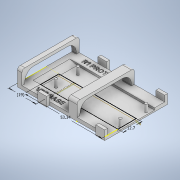
# Autodesk Inventor part: R1 Proto V10 Base
Saved by Autodesk Inventor 2021 (Build 250183000, 183)
## iProperties
Created: 2020-06-07
Part Number: R1 Proto V10 Base
Material: Generic
Document SubType Name: Modeling
Designer: andre
Density: 1 g/cm^3
Appearance: Default
Author: andre
## iProperties of the stored document _3DPrint.ipt
Created: 2020-06-07
Part Number: _3DPrint
Material: Generic
Document SubType Name: Modeling
Designer: andre
Density: 1 g/cm^3
Appearance: Default
Author: andre
Autodesk Inventor part; units mm, degrees
ref_plane "YZ Plane" through (0, 0, 0) normal (1, 0, 0) x (0, 1, 0)
ref_plane "XZ Plane" through (0, 0, 0) normal (0, 1, 0) x (-1, 0, 0)
ref_plane "XY Plane" through (0, 0, 0) normal (0, 0, 1) x (1, 0, 0)
sketch "Sketch1" plane through (0, 0, 0) normal (0, 1, 0) x (-1, 0, 0)
  line L0 (0, 0) -> (62, 0)
  line L1 (62, 0) -> (62, -19.7)
  line L2 (62, -19.7) -> (0, -19.7)
  line L3 (0, -19.7) -> (0, 0)
  dimension "d5" = 62
  dimension "d6" = 19.7
  constraints: 8 end point, 2 parallel, 1 horizontal, 1 perpendicular
  measures "d5" distance of L1.end L2.end
  measures "d6" distance of L0.end L1.end
extrude "Extrusion1" add sketch "Sketch1" along normal blind 2.4
sketch "Sketch2" plane through (0, 2.4, 0) normal (0, 1, 0) x (1, 0, 0)
  point P0 (0, 0)
sketch "Sketch3" plane through (-62, 0, 0) normal (0, 0, 1) x (1, 0, 0)
  line L0 (62, 2.4) -> (0, 2.4) projected
  line L1 (62, 0) -> (0, 0) projected
  line L2 (62, 2.4) -> (56, 2.4)
  line L3 (56, 2.4) -> (56, 0)
  line L4 (56, 0) -> (62, 0)
  line L5 (62, 0) -> (62, 2.4)
  line L6 (22, 2.4) -> (22, 0) construction
  line L7 (22, 2.4) -> (16, 2.4)
  line L8 (16, 2.4) -> (16, 0)
  line L9 (16, 0) -> (22, 0)
  line L10 (22, 0) -> (22, 2.4)
  point P0 (62, 0)
  point P1 (22, 0)
  dimension "d9" = 6
  dimension "d13" = 6
  dimension "d14" = 34
  constraints: 18 end point, 4 parallel, 4 point on line, 3 perpendicular, 2 horizontal
  measures "d9" distance of L4.end L3.end
  measures "d13" distance of L9.end L8.end
  measures "d14" distance between parallel lines of L3 L6
extrude "Extrusion2" add sketch "Sketch3" along normal blind 2 contours L5 L1 L3 L0 | L10 L1 L8 L0
ref_plane "Work Plane1" through (0, 0, -19.7) normal (0, 0, -1) x (-1, 0, 0)
sketch "Sketch4" plane through (0, 2.4, 0) normal (0, 1, 0) x (1, 0, 0)
  line L0 (-6, -2) -> (0, -2) projected
  line L1 (-6, -2) -> (0, -2)
  line L2 (0, -2) -> (0, 0)
  line L3 (0, 0) -> (-6, 0)
  line L4 (-6, 0) -> (-6, -2)
  line L5 (-46, -2) -> (-40, -2) projected
  line L6 (-40, 0) -> (-40, -2) projected
  line L7 (-46, -2) -> (-40, -2)
  line L8 (-40, -2) -> (-40, 0)
  line L9 (-40, 0) -> (-46, 0)
  line L10 (-46, 0) -> (-46, -2)
  constraints: 16 end point, 4 parallel, 2 horizontal, 2 perpendicular
extrude "Extrusion3" add sketch "Sketch4" along normal blind 4
sketch "Sketch5" plane through (0, 2.4, 0) normal (0, 1, 0) x (1, 0, 0)
  point P0 (0, 0)
sketch "Sketch6" plane through (0, 2.4, 0) normal (0, 1, 0) x (1, 0, 0)
  line L0 (0, 19.7) -> (-62, 19.7) projected
  line L1 (-40, 0) -> (-6, 0) projected
  line L2 (-21, 19.7) -> (-27, 19.7)
  line L3 (-27, 19.7) -> (-27, 0)
  line L4 (-27, 0) -> (-21, 0)
  line L5 (-21, 0) -> (-21, 19.7)
  line L6 (0, 19.7) -> (0, 0) projected
  dimension "d18" = 6
  dimension "d19" = 21
  constraints: 8 end point, 2 parallel, 2 point on line, 1 horizontal, 1 perpendicular
  measures "d18" distance of L4.end L3.end
  measures "d19" distance between parallel lines of L6 L5
extrude "Extrusion4" add sketch "Sketch6" along normal blind 9.6
sketch "Sketch7" plane through (-21, 2.4, 0) normal (1, 0, 0) x (0, 0, -1)
  point P0 (0, -2.4)
sketch "Sketch8" plane through (-21, 2.4, 0) normal (1, 0, 0) x (0, 0, -1)
  line L0 (19.7, 0) -> (19.7, 9.6) projected
  line L1 (19.7, 0) -> (2, 0)
  line L2 (2, 0) -> (2, 7.6)
  line L3 (2, 7.6) -> (19.7, 7.6)
  line L4 (19.7, 7.6) -> (19.7, 0)
  line L5 (0, 0) -> (0, 9.6) projected
  line L6 (19.7, 0) -> (0, 0) projected
  line L7 (0, 9.6) -> (19.7, 9.6) projected
  point P0 (0, -2.4)
  dimension "d22" = 19.7
  dimension "d23" = 9.6
  dimension "d24" = 17.7
  dimension "d25" = 7.6
  constraints: 8 end point, 2 parallel, 1 horizontal, 1 perpendicular
  measures "d22" distance between parallel lines of L0 L5
  measures "d23" distance between parallel lines of L6 L7
  measures "d24" distance between parallel lines of L0 L2
  measures "d25" distance between parallel lines of L1 L3
extrude "Extrusion5" cut sketch "Sketch8" against normal blind 37.6 contours L1 L2 L3 L0
sketch "Sketch9" plane through (0, 2.4, 0) normal (0, 1, 0) x (1, 0, 0)
  line L0 (-40, 0) -> (-46, 0) construction
  line L1 (-43, 0) -> (-43, 19.7) construction
  line L2 (0, 19.7) -> (-62, 19.7) construction
  line L3 (-62, 19.7) -> (-62, 0) projected
  point P0 (0, 0)
  dimension "d30" = 19
  constraints: 2 end point, 1 midpoint, 1 point on line, 1 vertical
  measures "d30" distance between parallel lines of L3 L1
ref_plane "Work Plane2" through (-43, 0, -19.7) normal (-1, 0, 0) x (0, 0, 1)
mirror "Mirror2" about plane through (-43, 0, -19.7) normal (-1, 0, 0) of "Extrusion4", "Extrusion5"
sketch "Sketch12" plane through (0, 2.4, 0) normal (0, 1, 0) x (1, 0, 0)
  line L0 (0, 19.7) -> (0, -2) projected
  line L1 (0, 19.7) -> (-53.34, 19.7)
  line L2 (-53.34, 19.7) -> (-53.34, 7)
  line L3 (-53.34, 7) -> (0, 7)
  line L4 (0, 7) -> (0, 19.7)
  point P0 (0, 0)
  point P1 (0, 7)
  dimension "d41" = 53.34
  dimension "d42" = 12.7
  constraints: 8 end point, 2 parallel, 1 horizontal, 1 perpendicular
  measures "d41" distance between parallel lines of L2 L0
  measures "d42" distance between parallel lines of L1 L3
extrude "Extrusion8" cut sketch "Sketch12" against normal blind 1.4
fillet "Fillet3" radius 2 2 edges at (-62, 12, 0) (-24, 12, 0) curvature continuous yes
fillet "Fillet4" radius 7 2 edges at (-62, 10, -2) (-24, 10, -2) curvature continuous yes
sketch "Sketch13" plane through (0, 1, 0) normal (0, 1, 0) x (1, 0, 0)
  circle A0 centre (-1.9751, 10.81) radius 0.9
  circle A1 centre (-47.6951, 12.1417) radius 0.9
  line L0 (-53.34, 19.7) -> (0, 19.7) projected
  point P0 (0, 0)
  dimension "d48" = 1.8
  dimension "d49" = 1.8
  dimension "d50" = 45.72
  dimension "d51" = 8.89
  constraints: 2 centre point
  measures "d48" diameter of A0
  measures "d49" diameter of A1
  measures "d50" horizontal distance of A1.centre A0.centre
  measures "d51" distance from line of L0 A0.centre
extrude "Extrusion9" add sketch "Sketch13" along normal blind 5
mirror "Mirror3" about plane through (0, 0, -19.7) normal (0, 0, -1) of "Extrusion4", "Extrusion5", "Mirror2", "Fillet4", "Fillet3", "Extrusion1", "Extrusion3", "Extrusion2", "Extrusion9", "Extrusion8"
sketch "Sketch14" plane through (-62, 0, 0) normal (-1, 0, 0) x (0, 0, 1)
  line L0 (-58.5888, -16.4354) -> (8.8289, -16.4354)
  line L1 (8.8289, -16.4354) -> (8.8289, 25.7982)
  line L2 (8.8289, 25.7982) -> (-58.5888, 25.7982)
  line L3 (-58.5888, 25.7982) -> (-58.5888, -16.4354)
  point P0 (0, 0)
  constraints: 8 end point, 2 parallel, 1 horizontal, 1 perpendicular
extrude "Extrusion10" cut sketch "Sketch14" along normal blind 5
chamfer "Chamfer1" distance 5 distance2 1.4 1 edges at (-53.34, 2.4, -19.7) measured on face at (-53.84, 2.4, -19.7)
sketch "Sketch15" plane through (0, 2.4, 0) normal (0, 1, 0) x (1, 0, 0)
  line L0 (-57, 38.4) -> (-29, 38.4) construction
  line L1 (-29, 38.4) -> (-29, 33.4) construction
  line L2 (-29, 33.4) -> (-57, 33.4) construction
  line L3 (-57, 33.4) -> (-57, 38.4) construction
  line L4 (-59, 37.4) -> (-59, 2) projected
  line L5 (-27, 2) -> (-27, 37.4) projected
  line L6 (-59, 39.4) -> (-46, 39.4) projected
  line L7 (-58.34, 32.4) -> (0, 32.4) projected
  line L8 (-57, 6) -> (-29, 6) construction
  line L9 (-29, 6) -> (-29, 1) construction
  line L10 (-29, 1) -> (-57, 1) construction
  line L11 (-57, 1) -> (-57, 6) construction
  line L12 (0, 7) -> (-58.34, 7) projected
  line L13 (-59, 0) -> (-46, 0) projected
  spline S0 degree 2 poles (-51.0157, 2) (-50.8394, 2) (-50.6147, 2.1691) (-50.5495, 2.3527) knots 0 0 0 1 2 2 2
  line L14 (-50.5495, 2.3527) -> (-49.7307, 4.5556)
  spline S1 degree 2 poles (-49.7307, 4.5556) (-49.7017, 4.6377) (-49.7017, 4.7174) knots 0 0 0 1 1 1
  spline S2 degree 2 poles (-49.7017, 4.7174) (-49.7041, 4.8454) (-49.8732, 4.9976) (-50.0157, 5) knots 0 0 0 1 2 2 2
  spline S3 degree 2 poles (-50.0157, 5) (-50.1341, 5) (-50.279, 4.8865) (-50.3176, 4.7657) knots 0 0 0 1 2 2 2
  line L15 (-50.3176, 4.7657) -> (-50.9988, 2.6691)
  line L16 (-50.9988, 2.6691) -> (-51.0133, 2.6691)
  line L17 (-51.0133, 2.6691) -> (-51.6969, 4.7585)
  spline S4 degree 2 poles (-51.6969, 4.7585) (-51.7331, 4.8841) (-51.8853, 5) (-52.0085, 5) knots 0 0 0 1 2 2 2
  spline S5 degree 2 poles (-52.0085, 5) (-52.1558, 4.9976) (-52.3273, 4.8406) (-52.3297, 4.7101) knots 0 0 0 1 2 2 2
  spline S6 degree 2 poles (-52.3297, 4.7101) (-52.3297, 4.6232) (-52.3007, 4.5386) knots 0 0 0 1 1 1
  line L18 (-52.3007, 4.5386) -> (-51.4867, 2.3551)
  spline S7 degree 2 poles (-51.4867, 2.3551) (-51.4215, 2.1691) (-51.1944, 2) (-51.0157, 2) knots 0 0 0 1 2 2 2
  spline S8 degree 2 poles (-48.3708, 1.9952) (-48.2331, 1.9976) (-48.0713, 2.1618) (-48.0688, 2.3019) knots 0 0 0 1 2 2 2
  line L19 (-48.0688, 2.3019) -> (-48.0688, 4.6618)
  spline S9 degree 2 poles (-48.0688, 4.6618) (-48.0713, 4.8213) (-48.2524, 5.0024) (-48.4167, 5.0048) knots 0 0 0 1 2 2 2
  spline S10 degree 2 poles (-48.4167, 5.0048) (-48.5085, 5.0048) (-48.6751, 4.9589) (-48.779, 4.8889) knots 0 0 0 1 2 2 2
  line L20 (-48.779, 4.8889) -> (-49.3587, 4.4879)
  spline S11 degree 2 poles (-49.3587, 4.4879) (-49.4287, 4.4372) (-49.4915, 4.3285) (-49.4915, 4.2585) knots 0 0 0 1 2 2 2
  spline S12 degree 2 poles (-49.4915, 4.2585) (-49.4891, 4.1594) (-49.3708, 4.0411) (-49.2766, 4.0411) knots 0 0 0 1 2 2 2
  spline S13 degree 2 poles (-49.2766, 4.0411) (-49.2307, 4.0411) (-49.1558, 4.0652) (-49.1147, 4.0942) knots 0 0 0 1 2 2 2
  line L21 (-49.1147, 4.0942) -> (-48.6872, 4.3937)
  line L22 (-48.6872, 4.3937) -> (-48.6751, 4.3937)
  line L23 (-48.6751, 4.3937) -> (-48.6751, 2.3019)
  spline S14 degree 2 poles (-48.6751, 2.3019) (-48.6727, 2.1618) (-48.5085, 1.9976) (-48.3708, 1.9952) knots 0 0 0 1 2 2 2
  spline S15 degree 2 poles (-46.2597, 1.9734) (-45.8877, 1.9758) (-45.3563, 2.3478) (-45.0713, 3.0314) (-45.0688, 3.5072) knots 0 0 0 1 2 3 3 3
  spline S16 degree 2 poles (-45.0688, 3.5072) (-45.0713, 3.9807) (-45.3563, 4.6594) (-45.8901, 5.0242) (-46.2597, 5.0266) knots 0 0 0 1 2 3 3 3
  spline S17 degree 2 poles (-46.2597, 5.0266) (-46.6292, 5.0242) (-47.163, 4.657) (-47.4505, 3.9783) (-47.4505, 3.5048) knots 0 0 0 1 2 3 3 3
  spline S18 degree 2 poles (-47.4505, 3.5048) (-47.4505, 3.029) (-47.163, 2.3454) (-46.6316, 1.9758) (-46.2597, 1.9734) knots 0 0 0 1 2 3 3 3
  spline S19 degree 2 poles (-46.2597, 2.4638) (-46.5326, 2.4662) (-46.8273, 3) (-46.8297, 3.5048) knots 0 0 0 1 2 2 2
  spline S20 degree 2 poles (-46.8297, 3.5048) (-46.8273, 4.0048) (-46.5278, 4.5338) (-46.2597, 4.5362) knots 0 0 0 1 2 2 2
  spline S21 degree 2 poles (-46.2597, 4.5362) (-45.9891, 4.5338) (-45.692, 4.0048) (-45.6896, 3.5048) knots 0 0 0 1 2 2 2
  spline S22 degree 2 poles (-45.6896, 3.5048) (-45.692, 3) (-45.9867, 2.4662) (-46.2597, 2.4638) knots 0 0 0 1 2 2 2
  line L24 (-43.535, 2.0386) -> (-42.5471, 2.0386)
  spline S23 degree 2 poles (-42.5471, 2.0386) (-42.0737, 2.0435) (-41.5423, 2.4855) (-41.5374, 2.8744) knots 0 0 0 1 2 2 2
  spline S24 degree 2 poles (-41.5374, 2.8744) (-41.5423, 3.1691) (-41.9215, 3.5531) (-42.2258, 3.5821) knots 0 0 0 1 2 2 2
  line L25 (-42.2258, 3.5821) -> (-42.2258, 3.5966)
  spline S25 degree 2 poles (-42.2258, 3.5966) (-41.9867, 3.6377) (-41.6824, 3.9855) (-41.6775, 4.2319) knots 0 0 0 1 2 2 2
  spline S26 degree 2 poles (-41.6775, 4.2319) (-41.68, 4.57) (-42.1534, 4.9565) (-42.5688, 4.9589) knots 0 0 0 1 2 2 2
  line L26 (-42.5688, 4.9589) -> (-43.535, 4.9589)
  spline S27 degree 2 poles (-43.535, 4.9589) (-43.68, 4.9589) (-43.8394, 4.7923) (-43.8394, 4.6425) knots 0 0 0 1 2 2 2
  line L27 (-43.8394, 4.6425) -> (-43.8394, 2.3575)
  spline S28 degree 2 poles (-43.8394, 2.3575) (-43.8394, 2.2053) (-43.68, 2.0386) (-43.535, 2.0386) knots 0 0 0 1 2 2 2
  line L28 (-43.2283, 2.4952) -> (-43.2283, 3.343)
  line L29 (-43.2283, 3.343) -> (-42.7162, 3.343)
  spline S29 degree 2 poles (-42.7162, 3.343) (-42.4457, 3.3406) (-42.1606, 3.128) (-42.1606, 2.9227) knots 0 0 0 1 2 2 2
  spline S30 degree 2 poles (-42.1606, 2.9227) (-42.1606, 2.7126) (-42.4384, 2.4952) (-42.7041, 2.4952) knots 0 0 0 1 2 2 2
  line L30 (-42.7041, 2.4952) -> (-43.2283, 2.4952)
  line L31 (-43.2283, 3.744) -> (-43.2283, 4.5048)
  line L32 (-43.2283, 4.5048) -> (-42.7283, 4.5048)
  spline S31 degree 2 poles (-42.7283, 4.5048) (-42.5109, 4.5024) (-42.279, 4.3116) (-42.279, 4.1353) knots 0 0 0 1 2 2 2
  spline S32 degree 2 poles (-42.279, 4.1353) (-42.279, 3.9493) (-42.5447, 3.7464) (-42.7911, 3.744) knots 0 0 0 1 2 2 2
  line L33 (-42.7911, 3.744) -> (-43.2283, 3.744)
  spline S33 degree 2 poles (-40.994, 2) (-40.8732, 2) (-40.7258, 2.1304) (-40.6848, 2.2754) knots 0 0 0 1 2 2 2
  line L34 (-40.6848, 2.2754) -> (-40.5302, 2.7319)
  line L35 (-40.5302, 2.7319) -> (-39.4771, 2.7319)
  line L36 (-39.4771, 2.7319) -> (-39.3225, 2.2705)
  spline S34 degree 2 poles (-39.3225, 2.2705) (-39.2814, 2.128) (-39.1316, 2) (-39.0036, 2) knots 0 0 0 1 2 2 2
  spline S35 degree 2 poles (-39.0036, 2) (-38.8684, 2.0024) (-38.7017, 2.1594) (-38.6993, 2.2874) knots 0 0 0 1 2 2 2
  spline S36 degree 2 poles (-38.6993, 2.2874) (-38.6993, 2.3333) (-38.7162, 2.4227) (-38.7379, 2.4831) knots 0 0 0 1 2 2 2
  line L37 (-38.7379, 2.4831) -> (-39.5399, 4.6546)
  spline S37 degree 2 poles (-39.5399, 4.6546) (-39.6027, 4.8333) (-39.8273, 5) (-40.006, 5) knots 0 0 0 1 2 2 2
  spline S38 degree 2 poles (-40.006, 5) (-40.1775, 5) (-40.4022, 4.8309) (-40.465, 4.6546) knots 0 0 0 1 2 2 2
  line L38 (-40.465, 4.6546) -> (-41.2621, 2.4831)
  spline S39 degree 2 poles (-41.2621, 2.4831) (-41.2838, 2.4251) (-41.3031, 2.3261) (-41.3031, 2.2874) knots 0 0 0 1 2 2 2
  spline S40 degree 2 poles (-41.3031, 2.2874) (-41.3031, 2.1546) (-41.1389, 2.0024) (-40.994, 2) knots 0 0 0 1 2 2 2
  line L39 (-40.3973, 3.2053) -> (-40.0181, 4.401)
  line L40 (-40.0181, 4.401) -> (-40.0036, 4.401)
  line L41 (-40.0036, 4.401) -> (-39.6171, 3.2053)
  line L42 (-39.6171, 3.2053) -> (-40.3973, 3.2053)
  spline S41 degree 2 poles (-37.2597, 1.9903) (-36.7089, 1.9952) (-36.0882, 2.4879) (-36.0833, 2.9203) knots 0 0 0 1 2 2 2
  spline S42 degree 2 poles (-36.0833, 2.9203) (-36.0809, 3.2512) (-36.5085, 3.6473) (-36.9698, 3.7367) knots 0 0 0 1 2 2 2
  line L43 (-36.9698, 3.7367) -> (-37.279, 3.7995)
  spline S43 degree 2 poles (-37.279, 3.7995) (-37.535, 3.8502) (-37.7669, 4.0266) (-37.7645, 4.1594) knots 0 0 0 1 2 2 2
  spline S44 degree 2 poles (-37.7645, 4.1594) (-37.7597, 4.3237) (-37.4915, 4.5145) (-37.2621, 4.5169) knots 0 0 0 1 2 2 2
  spline S45 degree 2 poles (-37.2621, 4.5169) (-37.0737, 4.5169) (-36.7983, 4.3696) (-36.7258, 4.2053) knots 0 0 0 1 2 2 2
  spline S46 degree 2 poles (-36.7258, 4.2053) (-36.6751, 4.1111) (-36.535, 4.0242) (-36.4336, 4.0242) knots 0 0 0 1 2 2 2
  spline S47 degree 2 poles (-36.4336, 4.0242) (-36.3152, 4.0266) (-36.1751, 4.1594) (-36.1727, 4.2681) knots 0 0 0 1 2 2 2
  spline S48 degree 2 poles (-36.1727, 4.2681) (-36.1727, 4.3092) (-36.1848, 4.3744) (-36.1944, 4.4058) knots 0 0 0 1 2 2 2
  spline S49 degree 2 poles (-36.1944, 4.4058) (-36.2959, 4.6932) (-36.8563, 5.0072) (-37.2621, 5.0097) knots 0 0 0 1 2 2 2
  spline S50 degree 2 poles (-37.2621, 5.0097) (-37.5882, 5.0072) (-38.0906, 4.7874) (-38.3732, 4.3913) (-38.378, 4.1208) knots 0 0 0 1 2 3 3 3
  spline S51 degree 2 poles (-38.378, 4.1208) (-38.378, 3.7947) (-37.9457, 3.3792) (-37.5085, 3.2923) knots 0 0 0 1 2 2 2
  line L44 (-37.5085, 3.2923) -> (-37.1993, 3.2319)
  spline S52 degree 2 poles (-37.1993, 3.2319) (-36.9263, 3.1763) (-36.692, 2.9976) (-36.6944, 2.8551) knots 0 0 0 1 2 2 2
  spline S53 degree 2 poles (-36.6944, 2.8551) (-36.6993, 2.6908) (-36.9964, 2.4855) (-37.2452, 2.4831) knots 0 0 0 1 2 2 2
  spline S54 degree 2 poles (-37.2452, 2.4831) (-37.4577, 2.4807) (-37.7742, 2.6401) (-37.849, 2.8068) knots 0 0 0 1 2 2 2
  spline S55 degree 2 poles (-37.849, 2.8068) (-37.9022, 2.901) (-38.0374, 2.9855) (-38.1292, 2.9831) knots 0 0 0 1 2 2 2
  spline S56 degree 2 poles (-38.1292, 2.9831) (-38.25, 2.9831) (-38.3973, 2.8382) (-38.3998, 2.715) knots 0 0 0 1 2 2 2
  spline S57 degree 2 poles (-38.3998, 2.715) (-38.3998, 2.6739) (-38.3829, 2.5894) (-38.3659, 2.5507) knots 0 0 0 1 2 2 2
  spline S58 degree 2 poles (-38.3659, 2.5507) (-38.2766, 2.3068) (-37.7138, 1.9952) (-37.2597, 1.9903) knots 0 0 0 1 2 2 2
  line L45 (-35.407, 2.0386) -> (-34.0181, 2.0386)
  spline S59 degree 2 poles (-34.0181, 2.0386) (-33.8901, 2.0386) (-33.7428, 2.1715) (-33.7403, 2.2923) knots 0 0 0 1 2 2 2
  spline S60 degree 2 poles (-33.7403, 2.2923) (-33.7428, 2.4106) (-33.8925, 2.5435) (-34.0181, 2.5435) knots 0 0 0 1 2 2 2
  line L46 (-34.0181, 2.5435) -> (-35.1002, 2.5435)
  line L47 (-35.1002, 2.5435) -> (-35.1002, 3.2826)
  line L48 (-35.1002, 3.2826) -> (-34.0713, 3.2826)
  spline S61 degree 2 poles (-34.0713, 3.2826) (-33.9529, 3.2826) (-33.8176, 3.4058) (-33.8152, 3.5169) knots 0 0 0 1 2 2 2
  spline S62 degree 2 poles (-33.8152, 3.5169) (-33.8176, 3.6256) (-33.9553, 3.7512) (-34.0713, 3.7512) knots 0 0 0 1 2 2 2
  line L49 (-34.0713, 3.7512) -> (-35.1002, 3.7512)
  line L50 (-35.1002, 3.7512) -> (-35.1002, 4.4541)
  line L51 (-35.1002, 4.4541) -> (-34.0181, 4.4541)
  spline S63 degree 2 poles (-34.0181, 4.4541) (-33.8925, 4.4541) (-33.7428, 4.587) (-33.7403, 4.7053) knots 0 0 0 1 2 2 2
  spline S64 degree 2 poles (-33.7403, 4.7053) (-33.7428, 4.8261) (-33.8901, 4.9589) (-34.0181, 4.9589) knots 0 0 0 1 2 2 2
  line L52 (-34.0181, 4.9589) -> (-35.407, 4.9589)
  spline S65 degree 2 poles (-35.407, 4.9589) (-35.5519, 4.9589) (-35.7114, 4.7923) (-35.7114, 4.6425) knots 0 0 0 1 2 2 2
  line L53 (-35.7114, 4.6425) -> (-35.7114, 2.3575)
  spline S66 degree 2 poles (-35.7114, 2.3575) (-35.7114, 2.2053) (-35.5519, 2.0386) (-35.407, 2.0386) knots 0 0 0 1 2 2 2
  spline S67 degree 2 poles (-52.1534, 34.3952) (-52.0085, 34.3976) (-51.849, 34.5618) (-51.8466, 34.714) knots 0 0 0 1 2 2 2
  line L54 (-51.8466, 34.714) -> (-51.8466, 35.5063)
  line L55 (-51.8466, 35.5063) -> (-51.3273, 35.5063)
  line L56 (-51.3273, 35.5063) -> (-50.8418, 34.6271)
  spline S68 degree 2 poles (-50.8418, 34.6271) (-50.7717, 34.4966) (-50.6365, 34.3928) (-50.5302, 34.3952) knots 0 0 0 1 2 2 2
  spline S69 degree 2 poles (-50.5302, 34.3952) (-50.3949, 34.3976) (-50.2258, 34.5522) (-50.221, 34.6754) knots 0 0 0 1 2 2 2
  spline S70 degree 2 poles (-50.221, 34.6754) (-50.221, 34.7261) (-50.25, 34.8227) (-50.2862, 34.8855) knots 0 0 0 1 2 2 2
  line L57 (-50.2862, 34.8855) -> (-50.7089, 35.615)
  spline S71 degree 2 poles (-50.7089, 35.615) (-50.465, 35.7213) (-50.2065, 36.1512) (-50.2065, 36.429) knots 0 0 0 1 2 2 2
  spline S72 degree 2 poles (-50.2065, 36.429) (-50.2089, 36.8662) (-50.7548, 37.3541) (-51.2621, 37.3589) knots 0 0 0 1 2 2 2
  line L58 (-51.2621, 37.3589) -> (-52.1534, 37.3589)
  spline S73 degree 2 poles (-52.1534, 37.3589) (-52.2983, 37.3589) (-52.4577, 37.1923) (-52.4577, 37.0425) knots 0 0 0 1 2 2 2
  line L59 (-52.4577, 37.0425) -> (-52.4577, 34.714)
  spline S74 degree 2 poles (-52.4577, 34.714) (-52.4577, 34.5618) (-52.2983, 34.3976) (-52.1534, 34.3952) knots 0 0 0 1 2 2 2
  line L60 (-51.8466, 35.9507) -> (-51.8466, 36.8807)
  line L61 (-51.8466, 36.8807) -> (-51.3273, 36.8807)
  spline S75 degree 2 poles (-51.3273, 36.8807) (-51.0978, 36.8783) (-50.837, 36.6319) (-50.8345, 36.4169) knots 0 0 0 1 2 2 2
  spline S76 degree 2 poles (-50.8345, 36.4169) (-50.8345, 36.1971) (-51.0882, 35.9531) (-51.3225, 35.9507) knots 0 0 0 1 2 2 2
  line L62 (-51.3225, 35.9507) -> (-51.8466, 35.9507)
  spline S77 degree 2 poles (-48.8104, 34.3952) (-48.6727, 34.3976) (-48.5109, 34.5618) (-48.5085, 34.7019) knots 0 0 0 1 2 2 2
  line L63 (-48.5085, 34.7019) -> (-48.5085, 37.0618)
  spline S78 degree 2 poles (-48.5085, 37.0618) (-48.5109, 37.2213) (-48.692, 37.4024) (-48.8563, 37.4048) knots 0 0 0 1 2 2 2
  spline S79 degree 2 poles (-48.8563, 37.4048) (-48.9481, 37.4048) (-49.1147, 37.3589) (-49.2186, 37.2889) knots 0 0 0 1 2 2 2
  line L64 (-49.2186, 37.2889) -> (-49.7983, 36.8879)
  spline S80 degree 2 poles (-49.7983, 36.8879) (-49.8684, 36.8372) (-49.9312, 36.7285) (-49.9312, 36.6585) knots 0 0 0 1 2 2 2
  spline S81 degree 2 poles (-49.9312, 36.6585) (-49.9287, 36.5594) (-49.8104, 36.4411) (-49.7162, 36.4411) knots 0 0 0 1 2 2 2
  spline S82 degree 2 poles (-49.7162, 36.4411) (-49.6703, 36.4411) (-49.5954, 36.4652) (-49.5543, 36.4942) knots 0 0 0 1 2 2 2
  line L65 (-49.5543, 36.4942) -> (-49.1268, 36.7937)
  line L66 (-49.1268, 36.7937) -> (-49.1147, 36.7937)
  line L67 (-49.1147, 36.7937) -> (-49.1147, 34.7019)
  spline S83 degree 2 poles (-49.1147, 34.7019) (-49.1123, 34.5618) (-48.9481, 34.3976) (-48.8104, 34.3952) knots 0 0 0 1 2 2 2
  spline S84 degree 2 poles (-46.692, 34.4) (-46.5471, 34.4024) (-46.3877, 34.5667) (-46.3853, 34.7188) knots 0 0 0 1 2 2 2
  line L68 (-46.3853, 34.7188) -> (-46.3853, 35.3589)
  line L69 (-46.3853, 35.3589) -> (-45.8394, 35.3589)
  spline S85 degree 2 poles (-45.8394, 35.3589) (-45.5302, 35.3614) (-45.0616, 35.6101) (-44.7983, 36.057) (-44.7983, 36.3589) knots 0 0 0 1 2 3 3 3
  spline S86 degree 2 poles (-44.7983, 36.3589) (-44.7983, 36.6609) (-45.0543, 37.1101) (-45.5085, 37.3565) (-45.8104, 37.3589) knots 0 0 0 1 2 3 3 3
  line L70 (-45.8104, 37.3589) -> (-46.692, 37.3589)
  spline S87 degree 2 poles (-46.692, 37.3589) (-46.837, 37.3589) (-46.9964, 37.1923) (-46.9964, 37.0425) knots 0 0 0 1 2 2 2
  line L71 (-46.9964, 37.0425) -> (-46.9964, 34.7188)
  spline S88 degree 2 poles (-46.9964, 34.7188) (-46.9964, 34.5667) (-46.837, 34.4024) (-46.692, 34.4) knots 0 0 0 1 2 2 2
  line L72 (-46.3853, 35.8372) -> (-46.3853, 36.8758)
  line L73 (-46.3853, 36.8758) -> (-45.9722, 36.8758)
  spline S89 degree 2 poles (-45.9722, 36.8758) (-45.7065, 36.8734) (-45.4215, 36.6077) (-45.4191, 36.3565) knots 0 0 0 1 2 2 2
  spline S90 degree 2 poles (-45.4191, 36.3565) (-45.4215, 36.1053) (-45.7089, 35.8396) (-45.9722, 35.8372) knots 0 0 0 1 2 2 2
  line L74 (-45.9722, 35.8372) -> (-46.3853, 35.8372)
  spline S91 degree 2 poles (-44.1316, 34.3952) (-43.9867, 34.3976) (-43.8273, 34.5618) (-43.8249, 34.714) knots 0 0 0 1 2 2 2
  line L75 (-43.8249, 34.714) -> (-43.8249, 35.5063)
  line L76 (-43.8249, 35.5063) -> (-43.3056, 35.5063)
  line L77 (-43.3056, 35.5063) -> (-42.82, 34.6271)
  spline S92 degree 2 poles (-42.82, 34.6271) (-42.75, 34.4966) (-42.6147, 34.3928) (-42.5085, 34.3952) knots 0 0 0 1 2 2 2
  spline S93 degree 2 poles (-42.5085, 34.3952) (-42.3732, 34.3976) (-42.2041, 34.5522) (-42.1993, 34.6754) knots 0 0 0 1 2 2 2
  spline S94 degree 2 poles (-42.1993, 34.6754) (-42.1993, 34.7261) (-42.2283, 34.8227) (-42.2645, 34.8855) knots 0 0 0 1 2 2 2
  line L78 (-42.2645, 34.8855) -> (-42.6872, 35.615)
  spline S95 degree 2 poles (-42.6872, 35.615) (-42.4432, 35.7213) (-42.1848, 36.1512) (-42.1848, 36.429) knots 0 0 0 1 2 2 2
  spline S96 degree 2 poles (-42.1848, 36.429) (-42.1872, 36.8662) (-42.7331, 37.3541) (-43.2403, 37.3589) knots 0 0 0 1 2 2 2
  line L79 (-43.2403, 37.3589) -> (-44.1316, 37.3589)
  spline S97 degree 2 poles (-44.1316, 37.3589) (-44.2766, 37.3589) (-44.436, 37.1923) (-44.436, 37.0425) knots 0 0 0 1 2 2 2
  line L80 (-44.436, 37.0425) -> (-44.436, 34.714)
  spline S98 degree 2 poles (-44.436, 34.714) (-44.436, 34.5618) (-44.2766, 34.3976) (-44.1316, 34.3952) knots 0 0 0 1 2 2 2
  line L81 (-43.8249, 35.9507) -> (-43.8249, 36.8807)
  line L82 (-43.8249, 36.8807) -> (-43.3056, 36.8807)
  spline S99 degree 2 poles (-43.3056, 36.8807) (-43.0761, 36.8783) (-42.8152, 36.6319) (-42.8128, 36.4169) knots 0 0 0 1 2 2 2
  spline S100 degree 2 poles (-42.8128, 36.4169) (-42.8128, 36.1971) (-43.0664, 35.9531) (-43.3007, 35.9507) knots 0 0 0 1 2 2 2
  line L83 (-43.3007, 35.9507) -> (-43.8249, 35.9507)
  spline S101 degree 2 poles (-40.4674, 34.3903) (-40.0326, 34.3928) (-39.4022, 34.7575) (-39.0616, 35.4314) (-39.0592, 35.8976) knots 0 0 0 1 2 3 3 3
  spline S102 degree 2 poles (-39.0592, 35.8976) (-39.0616, 36.3662) (-39.4022, 37.0425) (-40.0326, 37.4072) (-40.4674, 37.4097) knots 0 0 0 1 2 3 3 3
  spline S103 degree 2 poles (-40.4674, 37.4097) (-40.9022, 37.4072) (-41.5326, 37.0425) (-41.8732, 36.3662) (-41.8756, 35.8976) knots 0 0 0 1 2 3 3 3
  spline S104 degree 2 poles (-41.8756, 35.8976) (-41.8732, 35.4314) (-41.5326, 34.7575) (-40.9022, 34.3928) (-40.4674, 34.3903) knots 0 0 0 1 2 3 3 3
  spline S105 degree 2 poles (-40.4674, 34.9) (-40.8321, 34.9048) (-41.2476, 35.4338) (-41.2524, 35.8976) knots 0 0 0 1 2 2 2
  spline S106 degree 2 poles (-41.2524, 35.8976) (-41.2476, 36.3638) (-40.8297, 36.8952) (-40.4674, 36.9) knots 0 0 0 1 2 2 2
  spline S107 degree 2 poles (-40.4674, 36.9) (-40.1051, 36.8952) (-39.6872, 36.3638) (-39.6848, 35.8976) knots 0 0 0 1 2 2 2
  spline S108 degree 2 poles (-39.6848, 35.8976) (-39.6872, 35.4338) (-40.1051, 34.9048) (-40.4674, 34.9) knots 0 0 0 1 2 2 2
  spline S109 degree 2 poles (-37.663, 34.4) (-37.5181, 34.4024) (-37.3587, 34.5667) (-37.3563, 34.7188) knots 0 0 0 1 2 2 2
  line L84 (-37.3563, 34.7188) -> (-37.3563, 36.8541)
  line L85 (-37.3563, 36.8541) -> (-36.7524, 36.8541)
  spline S110 degree 2 poles (-36.7524, 36.8541) (-36.6268, 36.8541) (-36.4795, 36.987) (-36.4771, 37.1053) knots 0 0 0 1 2 2 2
  spline S111 degree 2 poles (-36.4771, 37.1053) (-36.4771, 37.2261) (-36.6268, 37.3589) (-36.7524, 37.3589) knots 0 0 0 1 2 2 2
  line L86 (-36.7524, 37.3589) -> (-38.5713, 37.3589)
  spline S112 degree 2 poles (-38.5713, 37.3589) (-38.6993, 37.3589) (-38.8466, 37.2261) (-38.849, 37.1053) knots 0 0 0 1 2 2 2
  spline S113 degree 2 poles (-38.849, 37.1053) (-38.8466, 36.987) (-38.6969, 36.8541) (-38.5713, 36.8541) knots 0 0 0 1 2 2 2
  line L87 (-38.5713, 36.8541) -> (-37.9674, 36.8541)
  line L88 (-37.9674, 36.8541) -> (-37.9674, 34.7188)
  spline S114 degree 2 poles (-37.9674, 34.7188) (-37.9674, 34.5667) (-37.808, 34.4024) (-37.663, 34.4) knots 0 0 0 1 2 2 2
  spline S115 degree 2 poles (-34.8563, 34.3903) (-34.4215, 34.3928) (-33.7911, 34.7575) (-33.4505, 35.4314) (-33.4481, 35.8976) knots 0 0 0 1 2 3 3 3
  spline S116 degree 2 poles (-33.4481, 35.8976) (-33.4505, 36.3662) (-33.7911, 37.0425) (-34.4215, 37.4072) (-34.8563, 37.4097) knots 0 0 0 1 2 3 3 3
  spline S117 degree 2 poles (-34.8563, 37.4097) (-35.2911, 37.4072) (-35.9215, 37.0425) (-36.2621, 36.3662) (-36.2645, 35.8976) knots 0 0 0 1 2 3 3 3
  spline S118 degree 2 poles (-36.2645, 35.8976) (-36.2621, 35.4314) (-35.9215, 34.7575) (-35.2911, 34.3928) (-34.8563, 34.3903) knots 0 0 0 1 2 3 3 3
  spline S119 degree 2 poles (-34.8563, 34.9) (-35.221, 34.9048) (-35.6365, 35.4338) (-35.6413, 35.8976) knots 0 0 0 1 2 2 2
  spline S120 degree 2 poles (-35.6413, 35.8976) (-35.6365, 36.3638) (-35.2186, 36.8952) (-34.8563, 36.9) knots 0 0 0 1 2 2 2
  spline S121 degree 2 poles (-34.8563, 36.9) (-34.494, 36.8952) (-34.0761, 36.3638) (-34.0737, 35.8976) knots 0 0 0 1 2 2 2
  spline S122 degree 2 poles (-34.0737, 35.8976) (-34.0761, 35.4338) (-34.494, 34.9048) (-34.8563, 34.9) knots 0 0 0 1 2 2 2
  point P0 (0, 0)
  dimension "d59" = 2
  dimension "d60" = 2
  dimension "d61" = 1
  dimension "d62" = 1
  dimension "d63" = 1
  dimension "d64" = 1
  dimension "d65" = 2
  dimension "d66" = 2
  constraints: 4 other
  measures "d59" distance between parallel lines of L4 L3
  measures "d60" distance between parallel lines of L5 L1
  measures "d61" distance between parallel lines of L6 L0
  measures "d62" distance between parallel lines of L7 L2
  measures "d63" distance between parallel lines of L12 L8
  measures "d64" distance between parallel lines of L13 L10
  measures "d65" distance between parallel lines of L4 L11
  measures "d66" distance between parallel lines of L5 L9
extrude "Extrusion11" cut sketch "Sketch15" against normal blind 1
equation "\"d49\" = d48"
equation "\"d60\" = d59"
equation "\"d62\" = d61"
equation "\"d63\" = d61"
equation "\"d64\" = d61"
equation "\"d65\" = d59"
equation "\"d66\" = d59"
equation "\"d29\" = -d30"
body "Solid1"
